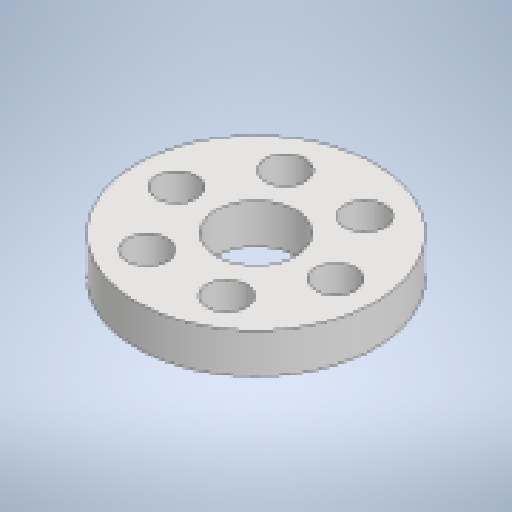
# Autodesk Inventor part: Plowette - Mount
Saved by Autodesk Inventor 2023.2 (Build 272271000, 271)
## iProperties
Created: 2023-04-05
Part Number: Plowette - Mount
Material: UHMW, White
Document SubType Name: Modeling
Designer: Nathan Cai
Density: 0.94 g/cm^3
Appearance: Smooth - White
Author: Nathan Cai
Autodesk Inventor part; units mm, degrees
ref_plane "YZ Plane" through (0, 0, 0) normal (1, 0, 0) x (0, 1, 0)
ref_plane "XZ Plane" through (0, 0, 0) normal (0, 1, 0) x (-1, 0, 0)
ref_plane "XY Plane" through (0, 0, 0) normal (0, 0, 1) x (1, 0, 0)
sketch "Sketch1" plane through (0, 0, 0) normal (0, 1, 0) x (-1, 0, 0)
  circle A0 centre (0, 0) radius 6.35 construction
  circle A1 centre (0, 0) radius 3.175
  line L0 (0, 0) -> (6.35, 0) construction
  circle A2 centre (6.35, 0) radius 1.5875
  circle A3 centre (3.175, 5.4993) radius 1.5875
  circle A4 centre (-3.175, 5.4993) radius 1.5875
  circle A5 centre (-6.35, 0) radius 1.5875
  circle A6 centre (-3.175, -5.4993) radius 1.5875
  circle A7 centre (3.175, -5.4993) radius 1.5875
  circle A8 centre (0, 0) radius 9.525
  dimension "d0" = 12.7
  dimension "d1" = 6.35
  dimension "d2" = 3.175
  dimension "d5" = 360
  dimension "d7" = 19.05
  constraints: 8 centre point, 4 coincident, 2 end point, 1 horizontal, 1 horizontal alignment, 15 other
  measures "d1" diameter of A1
  measures "d2" diameter of A2
  measures "d7" diameter of A8
extrude "Extrusion1" add sketch "Sketch1" along normal blind 1.5875
sketch "Sketch2" plane through (0, 1.5875, 0) normal (0, 1, 0) x (1, 0, 0)
  circle A0 centre (0, 0) radius 9.525 construction
  circle A1 centre (-3.175, 5.4993) radius 1.5875 projected
  circle A2 centre (3.175, 5.4993) radius 1.5875 projected
  circle A3 centre (6.35, 0) radius 1.5875 projected
  circle A4 centre (3.175, -5.4993) radius 1.5875 projected
  circle A5 centre (-3.175, -5.4993) radius 1.5875 projected
  circle A6 centre (-6.35, 0) radius 1.5875 projected
  circle A7 centre (0, 0) radius 3.175 projected
  line L0 (0, 0) -> (0, -25.4) construction
  line L1 (-9.525, 0) -> (-9.525, -25.4)
  line L2 (9.525, -25.4) -> (9.525, 0)
  arc A8 (9.525, 0) -> (-9.525, 0) centre (0, 0) ccw
  arc A9 (-9.525, -25.4) -> (9.525, -25.4) centre (0, -25.4) ccw
  circle A10 centre (0, 0) radius 9.525 projected
  point P0 (0, -12.7)
  dimension "d10" = 25.4
  constraints: 8 end point, 4 point on circle, 4 tangent, 2 centre point, 1 horizontal alignment, 1 midpoint, 1 parallel, 1 vertical, 1 other
  measures "d10" distance of L0.start L0.end
extrude "Extrusion2" add sketch "Sketch2" along normal blind 3.175
body "Solid1"
